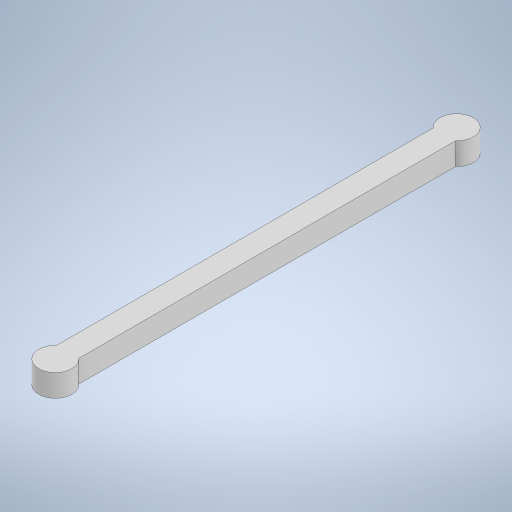
# Autodesk Inventor part: link_wp2kp
Saved by Autodesk Inventor 2024.3 (Build 283343000, 343)
## iProperties
Created: 2025-01-18
Part Number: link_wp2kp
Material: 一般
Document SubType Name: Modeling
Designer: yuu53
Density: 1 g/cm^3
Appearance: 既定
Author: yuu53
Autodesk Inventor part; units mm, degrees
ref_plane "YZ Plane" through (0, 0, 0) normal (1, 0, 0) x (0, 1, 0)
ref_plane "XZ Plane" through (0, 0, 0) normal (0, 1, 0) x (-1, 0, 0)
ref_plane "XY Plane" through (0, 0, 0) normal (0, 0, 1) x (1, 0, 0)
sketch "スケッチ1" plane through (0, 0, 0) normal (0, 1, 0) x (-1, 0, 0)
  circle A0 centre (0, 90) radius 7.5
  circle A1 centre (0, -90) radius 7.5
  line L0 (5, 90) -> (-5, 90)
  line L1 (-5, 90) -> (-5, -90)
  line L2 (-5, -90) -> (5, -90)
  line L3 (5, -90) -> (5, 90)
  point P0 (0, 0)
  point P1 (0, 90)
  point P2 (5, -84.4098)
  point P3 (5, 84.4098)
  point P4 (-5, 84.4098)
  point P5 (-5, -84.4098)
  dimension "d0" = 180
  dimension "d1" = 5
  dimension "d2" = 10
  dimension "d3" = 90
  dimension "d4" = 0
  dimension "d5" = 0
  dimension "d6" = 15
  dimension "d7" = 15
  constraints: 8 end point, 2 centre point, 2 midpoint, 2 parallel, 1 horizontal, 1 perpendicular
  measures "d0" distance of L0.end L1.end
  measures "d1" distance from line of L1 point (0, 0)
  measures "d2" distance of L0.start L0.end
  measures "d3" distance of point (0, 0) point (0, -90)
  measures "d4" distance of point (0, 90) A0.centre
  measures "d5" distance of point (0, -90) A1.centre
  measures "d6" diameter of A1
  measures "d7" diameter of A0
extrude "押し出し1" add sketch "スケッチ1" along normal blind 5 and the other way blind 5
